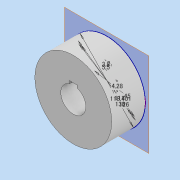
# Autodesk Inventor part: gear2
Saved by Autodesk Inventor 2022 (Build 260153000, 153)
## iProperties
Created: 2023-12-21
Part Number: gear2
Material: 一般
Document SubType Name: Modeling
Designer: ktamu
Density: 1 g/cm^3
Appearance: 既定
Author: ktamu
Autodesk Inventor part; units mm, degrees
ref_plane "YZ Plane" through (0, 0, 0) normal (1, 0, 0) x (0, 1, 0)
ref_plane "XZ Plane" through (0, 0, 0) normal (0, 1, 0) x (-1, 0, 0)
ref_plane "XY Plane" through (0, 0, 0) normal (0, 0, 1) x (1, 0, 0)
sketch "スケッチ1" plane through (0, 0, 0) normal (0, 0, 1) x (1, 0, 0)
  circle A0 centre (0, 0) radius 69
  arc A1 (-6.6994, 21.4795) -> (7, 21.3834) centre (0, 0) ccw
  line L0 (0, 22.5) -> (0, 17)
  line L1 (0, 22.5) -> (0, 26.3)
  line L2 (0, 26.3) -> (7, 26.3)
  line L3 (7, 26.3) -> (7, 21.3834)
  line L4 (7, 17) -> (0, 17)
  line L5 (-6.6994, 21.4795) -> (-6.6994, 26.3)
  line L6 (-6.6994, 26.3) -> (0, 26.3)
  circle A2 centre (0, 0) radius 63 construction
  circle A3 centre (0, 0) radius 55.5 construction
  circle A4 centre (0, 0) radius 59.2005 construction
  line L7 (0, 0) -> (59.0354, 4.4182)
  line L8 (0, 0) -> (63, 0) construction
  line L9 (68.4937, 8.3432) -> (69.7595, 0)
  line L10 (55.4029, 3.282) -> (55.5, 0)
  line L11 (44.4457, 0) -> (43.0115, 0)
  circle A5 centre (0, 0) radius 55.5 construction
  line L12 (68.4937, -8.3432) -> (69.7595, 0)
  line L13 (55.5, 0) -> (55.4029, -3.282)
  line L14 (0, 0) -> (22.4606, -1.3305)
  line L15 (55.4029, -3.282) -> (59.0929, -3.5681)
  line L16 (0, 0) -> (22.4606, 1.3305)
  line L17 (55.4029, 3.282) -> (59.0929, 3.5681)
  dimension "d0" = 138
  dimension "d1" = 45
  dimension "d2" = 5.5
  dimension "d3" = 3.8
  dimension "d4" = 7
  dimension "d7" = 126
  dimension "d8" = 111
  dimension "d9" = 118.401
  dimension "d12" = 4.28
  constraints: 36 end point, 10 point on circle, 6 coincident, 5 centre point, 5 point on line, 3 horizontal, 3 perpendicular, 2 vertical, 1 collinear, 10 other
  measures "d1" diameter of A1
  measures "d2" distance of L0.end L0.start
  measures "d3" distance of L0.start L1.end
  measures "d4" distance of L1.end L2.end
  measures "d7" diameter of A2
  measures "d8" diameter of A3
  measures "d9" diameter of A4
  measures "d12" angle of L8 L7
extrude "押し出し1" add sketch "スケッチ1" along normal blind 60 contours A0
sketch "スケッチ2" plane through (0, 0, 0) normal (1, 0, 0) x (0, 1, 0)
  point P0 (0, 0)
ref_plane "作業平面1" through (0, 0, 0) normal (0, 0, -1) x (-1, 0, 0)
sketch "スケッチ3" plane through (0, 0, 0) normal (0, 0, -1) x (-1, 0, 0)
  line L0 (-55.4145, -3.3023) -> (-55.4145, 3.2937)
  line L1 (-55.4145, 3.2937) -> (-59.0906, 3.5877)
  point P0 (0, 0)
  constraints: 4 end point, 1 vertical
